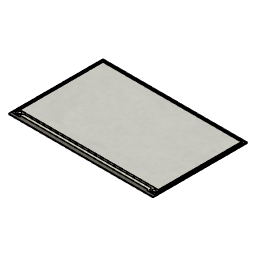
Openbook complet (Autodesk Fusion 360 archive; units mm, degrees)
design "Display"
Autodesk Fusion 360 part; units mm, degrees
sketch "Sketch1" plane through (0, 0, 0) normal (0, 0, 1) x (1, 0, 0)
  line L0 (0, 0) -> (170.2, 0)
  line L1 (170.2, 0) -> (170.2, 111.2)
  line L2 (170.2, 111.2) -> (0, 111.2)
  line L3 (0, 111.2) -> (0, 0)
  dimension "d1" = 170.2
  dimension "d2" = 111.2
  constraint horizontal L0
  constraint vertical L1
  constraint horizontal L2
  constraint vertical L3
  constraint coincident L0.start L3.end
  measures "d1" distance of L0.start L0.end
  measures "d2" distance of L0.end L1.end
extrude "Extrude1" add sketch "Sketch1" along normal blind 0.07 makes body 1
sketch "Sketch2" plane through (0, 0, 0.07) normal (0, 0, 1) x (-1, 0, 0)
  line L0 (0, -111.2) -> (0, 0)
  line L1 (0, 0) -> (-170.2, 0)
  line L2 (-170.2, 0) -> (-170.2, -111.2)
  line L3 (-170.2, -111.2) -> (0, -111.2)
  line L4 (-1.2, -110) -> (-169, -110)
  line L5 (-169, -110) -> (-169, -2.91)
  line L6 (-169, -2.91) -> (-1.2, -2.91)
  line L7 (-1.2, -2.91) -> (-1.2, -110)
  dimension "d6" = 167.8
  dimension "d7" = 107.09
  constraint horizontal L4
  constraint vertical L5
  constraint horizontal L6
  constraint vertical L7
  measures "d6" distance of L4.start L4.end
  measures "d7" distance of L4.start L6.end
extrude "Extrude2" add sketch "Sketch2" along normal blind 0.06 separate body contours L4 L5 L6 L7 makes body 2
sketch "Sketch3" plane through (0, 0, 0.13) normal (0, 0, 1) x (-1, 0, 0)
  line L0 (-1.2, -2.91) -> (-169, -2.91)
  line L1 (-169, -2.91) -> (-169, -110)
  line L2 (-169, -110) -> (-1.2, -110)
  line L3 (-1.2, -110) -> (-1.2, -2.91)
  line L4 (-169, -2.91) -> (-160, -2.91)
  spline S0 degree 5 poles (-10.2, -2.91) (-10.2046, -2.9696) (-10.2134, -3.086) (-10.226, -3.2529) (-10.2412, -3.4594) (-10.258, -3.6905) (-10.2727, -3.8935) (-10.2862, -4.0679) (-10.3001, -4.2136) (-10.3166, -4.3314) (-10.3392, -4.4237) (-10.3718, -4.4938) (-10.4184, -4.5453) (-10.4822, -4.5814) (-10.565, -4.6046) (-10.6676, -4.6167) (-10.7655, -4.6183) (-10.8476, -4.6151) (-10.9061, -4.6111) (-10.9364, -4.6086) knots 0 0 0 0 0 0 0.066667 0.133333 0.2 0.266667 0.333333 0.4 0.466667 0.533333 0.6 0.666667 0.733333 0.8 0.866667 0.933333 1 1 1 1 1 1
  spline S1 degree 5 poles (-160, -2.91) (-160.0003, -2.9773) (-159.9997, -3.108) (-159.9949, -3.2923) (-159.9808, -3.5144) (-159.9499, -3.7519) (-159.9052, -3.9484) (-159.8458, -4.1039) (-159.7711, -4.2198) (-159.6803, -4.3001) (-159.5732, -4.351) (-159.4493, -4.3798) (-159.3085, -4.3938) (-159.1511, -4.3991) (-158.9775, -4.3996) (-158.7883, -4.3978) (-158.625, -4.3954) (-158.4959, -4.3933) (-158.407, -4.3917) (-158.3618, -4.3909) knots 0 0 0 0 0 0 0.066667 0.133333 0.2 0.266667 0.333333 0.4 0.466667 0.533333 0.6 0.666667 0.733333 0.8 0.866667 0.933333 1 1 1 1 1 1
  line L5 (-10.9364, -4.6086) -> (-158.3618, -4.3909)
  point P0 (-10.3, -4.2)
  point P1 (-10.4443, -4.5566)
  point P2 (-159.805, -4.1594)
  point P3 (-159.3149, -4.3909)
  dimension "d10" = 9
  dimension "d11" = 9
  constraint horizontal L4
  constraint coincident L0.end L1.start
  measures "d10" distance of L0.start S0.start
  measures "d11" distance of L0.end L4.end
extrude "Extrude3" cut sketch "Sketch3" against normal blind 0.06 contours L0 S0 S1 L5 bodies 2
sketch "Sketch4" plane through (0, 0, 0.13) normal (0, 0, 1) x (-1, 0, 0)
  spline S0 degree 5 poles (-158.3618, -4.3909) (-158.407, -4.3917) (-158.4959, -4.3933) (-158.625, -4.3954) (-158.7883, -4.3978) (-158.9775, -4.3996) (-159.1511, -4.3991) (-159.3085, -4.3938) (-159.4493, -4.3798) (-159.5732, -4.351) (-159.6803, -4.3001) (-159.7711, -4.2198) (-159.8458, -4.1039) (-159.9052, -3.9484) (-159.9499, -3.7519) (-159.9808, -3.5144) (-159.9949, -3.2923) (-159.9997, -3.108) (-160.0003, -2.9773) (-160, -2.91) knots -1 -1 -1 -1 -1 -1 -0.933333 -0.866667 -0.8 -0.733333 -0.666667 -0.6 -0.533333 -0.466667 -0.4 -0.333333 -0.266667 -0.2 -0.133333 -0.066667 0 0 0 0 0 0
  line L0 (-160, -2.91) -> (-169, -2.91)
  line L1 (-169, -2.91) -> (-169, -110)
  line L2 (-169, -110) -> (-1.2, -110)
  line L3 (-1.2, -110) -> (-1.2, -2.91)
  line L4 (-1.2, -2.91) -> (-10.2, -2.91)
  spline S1 degree 5 poles (-10.2, -2.91) (-10.2046, -2.9696) (-10.2134, -3.086) (-10.226, -3.2529) (-10.2412, -3.4594) (-10.258, -3.6905) (-10.2727, -3.8935) (-10.2862, -4.0679) (-10.3001, -4.2136) (-10.3166, -4.3314) (-10.3392, -4.4237) (-10.3718, -4.4938) (-10.4184, -4.5453) (-10.4822, -4.5814) (-10.565, -4.6046) (-10.6676, -4.6167) (-10.7655, -4.6183) (-10.8476, -4.6151) (-10.9061, -4.6111) (-10.9364, -4.6086) knots 0 0 0 0 0 0 0.066667 0.133333 0.2 0.266667 0.333333 0.4 0.466667 0.533333 0.6 0.666667 0.733333 0.8 0.866667 0.933333 1 1 1 1 1 1
  line L5 (-10.9364, -4.6086) -> (-158.3618, -4.3909)
  line L6 (-2.7, -108.5) -> (-167.5, -108.5)
  line L7 (-167.5, -108.5) -> (-167.5, -4.41)
  line L8 (-167.5, -4.41) -> (-2.7, -4.41)
  line L9 (-2.7, -4.41) -> (-2.7, -108.5)
  dimension "d17" = 164.8
  dimension "d18" = 104.09
  constraint horizontal L6
  constraint vertical L7
  constraint horizontal L8
  constraint vertical L9
  measures "d17" distance of L6.start L6.end
  measures "d18" distance of L6.start L8.end
extrude "Extrude4" add sketch "Sketch4" along normal blind 0.16 separate body contours S1 L5 L6 L7 L8 L9 makes body 3
sketch "Sketch5" plane through (0, 0, 0.07) normal (0, 0, 1) x (-1, 0, 0)
  line L0 (0, -111.2) -> (0, 0)
  line L1 (0, 0) -> (-170.2, 0)
  line L2 (-170.2, 0) -> (-170.2, -111.2)
  line L3 (-170.2, -111.2) -> (0, -111.2)
  line L4 (0, -111.2) -> (-170.2, -111.2)
  line L5 (-170.2, -111.2) -> (-170.2, 0)
  line L6 (-170.2, 0) -> (0, 0)
  line L7 (0, 0) -> (0, -111.2)
  dimension "d21" = 170.2
  dimension "d22" = 111.2
  constraint horizontal L4
  constraint vertical L5
  constraint horizontal L6
  constraint vertical L7
  constraint coincident L0.start L3.end
  measures "d21" distance of L0.start L2.end
  measures "d22" distance of L0.start L0.end
extrude "Extrude5" add sketch "Sketch5" along normal blind 0.63 bodies 1
move_body "Move1" bodies 2 to x (1, 0, 0) y (0, 1, 0) z (0, 0, 1) at (0, 0, 0.7)
extrude "Extrude6" add 1 faces at (109.5206, 74.797, 0.83) along direction (0, 0, 1) blind 0.1 on bodies 2 bodies 2
move_body "Move2" bodies 3 to x (1, 0, 0) y (0, 1, 0) z (0, 0, 1) at (0, 0, 0.86)
sketch "Sketch6" plane through (0, 0, 1.15) normal (0, 0, 1) x (-1, 0, 0)
  spline S0 degree 5 poles (-10.339, -4.41) (-10.3395, -4.4117) (-10.3455, -4.4299) (-10.3581, -4.4622) (-10.3802, -4.5031) (-10.4184, -4.5453) (-10.4822, -4.5814) (-10.565, -4.6046) (-10.6676, -4.6167) (-10.7655, -4.6183) (-10.8476, -4.6151) (-10.9061, -4.6111) (-10.9364, -4.6086) knots 0.526762 0.526762 0.526762 0.526762 0.526762 0.526762 0.533333 0.6 0.666667 0.733333 0.8 0.866667 0.933333 1 1 1 1 1 1
  line L0 (-10.9364, -4.6086) -> (-145.4015, -4.41)
  line L1 (-145.4015, -4.41) -> (-167.5, -4.41)
  line L2 (-167.5, -4.41) -> (-167.5, -108.5)
  line L3 (-167.5, -108.5) -> (-2.7, -108.5)
  line L4 (-2.7, -108.5) -> (-2.7, -4.41)
  line L5 (-2.7, -4.41) -> (-10.339, -4.41)
  spline S1 degree 5 poles (-8.7, -4.41) (-8.707, -4.4556) (-8.7209, -4.5443) (-8.7408, -4.6698) (-8.7659, -4.8221) (-8.7948, -4.9867) (-8.8215, -5.125) (-8.8466, -5.237) (-8.8716, -5.3232) (-8.8985, -5.3859) (-8.9302, -5.4287) (-8.97, -5.4564) (-9.021, -5.4735) (-9.0857, -5.484) (-9.1653, -5.4907) (-9.2604, -5.4952) (-9.3487, -5.4977) (-9.4217, -5.499) (-9.4734, -5.4997) (-9.5, -5.5) knots 0 0 0 0 0 0 0.066667 0.133333 0.2 0.266667 0.333333 0.4 0.466667 0.533333 0.6 0.666667 0.733333 0.8 0.866667 0.933333 1 1 1 1 1 1
  spline S2 degree 5 poles (-161.5, -4.41) (-161.4999, -4.4539) (-161.4995, -4.5394) (-161.4982, -4.6608) (-161.4948, -4.8087) (-161.4879, -4.97) (-161.478, -5.1071) (-161.4646, -5.2198) (-161.4468, -5.3086) (-161.4236, -5.3751) (-161.3936, -5.4225) (-161.3554, -5.4547) (-161.3075, -5.4756) (-161.2488, -5.4889) (-161.179, -5.4968) (-161.0979, -5.501) (-161.0241, -5.5019) (-160.9639, -5.5014) (-160.9217, -5.5006) (-160.9, -5.5) knots 0 0 0 0 0 0 0.066667 0.133333 0.2 0.266667 0.333333 0.4 0.466667 0.533333 0.6 0.666667 0.733333 0.8 0.866667 0.933333 1 1 1 1 1 1
  line L6 (-160.9, -5.5) -> (-9.5, -5.5)
  point P0 (-8.8643, -5.2936)
  point P1 (-9.0307, -5.4733)
  point P2 (-161.451, -5.2805)
  point P3 (-161.2937, -5.4771)
  dimension "d27" = 6
  dimension "d29" = 6
  measures "d27" distance of L4.end S1.start
  measures "d29" distance of L1.end S2.start
extrude "Extrude7" cut sketch "Sketch6" against normal blind 0.16 contours S0 L0 L1 L5 S1 S2 L6 bodies 3
sketch "Sketch7" plane through (0, 0, 1.15) normal (0, 0, 1) x (-1, 0, 0)
  spline S0 degree 5 poles (-160.9, -5.5) (-160.9217, -5.5006) (-160.9639, -5.5014) (-161.0241, -5.5019) (-161.0979, -5.501) (-161.179, -5.4968) (-161.2488, -5.4889) (-161.3075, -5.4756) (-161.3554, -5.4547) (-161.3936, -5.4225) (-161.4236, -5.3751) (-161.4468, -5.3086) (-161.4646, -5.2198) (-161.478, -5.1071) (-161.4879, -4.97) (-161.4948, -4.8087) (-161.4982, -4.6608) (-161.4995, -4.5394) (-161.4999, -4.4539) (-161.5, -4.41) knots -1 -1 -1 -1 -1 -1 -0.933333 -0.866667 -0.8 -0.733333 -0.666667 -0.6 -0.533333 -0.466667 -0.4 -0.333333 -0.266667 -0.2 -0.133333 -0.066667 0 0 0 0 0 0
  line L0 (-161.5, -4.41) -> (-167.5, -4.41)
  line L1 (-167.5, -4.41) -> (-167.5, -108.5)
  line L2 (-167.5, -108.5) -> (-2.7, -108.5)
  line L3 (-2.7, -108.5) -> (-2.7, -4.41)
  line L4 (-2.7, -4.41) -> (-8.7, -4.41)
  spline S1 degree 5 poles (-8.7, -4.41) (-8.707, -4.4556) (-8.7209, -4.5443) (-8.7408, -4.6698) (-8.7659, -4.8221) (-8.7948, -4.9867) (-8.8215, -5.125) (-8.8466, -5.237) (-8.8716, -5.3232) (-8.8985, -5.3859) (-8.9302, -5.4287) (-8.97, -5.4564) (-9.021, -5.4735) (-9.0857, -5.484) (-9.1653, -5.4907) (-9.2604, -5.4952) (-9.3487, -5.4977) (-9.4217, -5.499) (-9.4734, -5.4997) (-9.5, -5.5) knots 0 0 0 0 0 0 0.066667 0.133333 0.2 0.266667 0.333333 0.4 0.466667 0.533333 0.6 0.666667 0.733333 0.8 0.866667 0.933333 1 1 1 1 1 1
  line L5 (-9.5, -5.5) -> (-160.9, -5.5)
  circle A0 centre (-6, -7) radius 1.8477
  circle A1 centre (-164.4622, -6.8748) radius 1.7327
sketch "Sketch8" plane through (0, 0, 1.15) normal (0, 0, 1) x (1, 0, 0)
  line L0 (2.7, 108.5) -> (3.5, 108.5)
  line L1 (3.5, 108.5) -> (3.5, 107.7)
  line L2 (3.5, 107.7) -> (2.7, 107.7)
  line L3 (2.7, 107.7) -> (2.7, 108.5)
  line L4 (3.5, 107.7) -> (166.7, 107.7)
  line L5 (166.7, 107.7) -> (166.7, 9.78)
  line L6 (166.7, 9.78) -> (3.5, 9.78)
  line L7 (3.5, 9.78) -> (3.5, 107.7)
  dimension "d36" = 0.8
  dimension "d37" = 0.8
  dimension "d38" = 163.2
  dimension "d39" = 97.92
  constraint horizontal L0
  constraint vertical L1
  constraint horizontal L2
  constraint vertical L3
  constraint horizontal L4
  constraint vertical L5
  constraint horizontal L6
  constraint vertical L7
  measures "d36" distance of L0.start L0.end
  measures "d37" distance of L0.start L2.end
  measures "d38" distance of L1.end L4.end
  measures "d39" distance of L1.end L6.end
extrude "Extrude8" cut sketch "Sketch7" against normal blind 0.08 contours A0 | A1 bodies 3
extrude "Extrude9" add sketch "Sketch8" along normal blind 0.16 separate body contours L4 L5 L6 L7 makes body 4
sketch "Sketch9" plane through (0, 0, 1.15) normal (0, 0, 1) x (-1, 0, 0)
  circle A0 centre (-6, -7) radius 1.8477
  circle A1 centre (-164.4622, -6.8748) radius 1.7327
  spline S0 degree 5 poles (-160.9, -5.5) (-160.9217, -5.5006) (-160.9639, -5.5014) (-161.0241, -5.5019) (-161.0979, -5.501) (-161.179, -5.4968) (-161.2488, -5.4889) (-161.3075, -5.4756) (-161.3554, -5.4547) (-161.3936, -5.4225) (-161.4236, -5.3751) (-161.4468, -5.3086) (-161.4646, -5.2198) (-161.478, -5.1071) (-161.4879, -4.97) (-161.4948, -4.8087) (-161.4982, -4.6608) (-161.4995, -4.5394) (-161.4999, -4.4539) (-161.5, -4.41) knots -1 -1 -1 -1 -1 -1 -0.933333 -0.866667 -0.8 -0.733333 -0.666667 -0.6 -0.533333 -0.466667 -0.4 -0.333333 -0.266667 -0.2 -0.133333 -0.066667 0 0 0 0 0 0
  line L0 (-161.5, -4.41) -> (-167.5, -4.41)
  line L1 (-167.5, -4.41) -> (-167.5, -108.5)
  line L2 (-167.5, -108.5) -> (-2.7, -108.5)
  line L3 (-2.7, -108.5) -> (-2.7, -4.41)
  line L4 (-2.7, -4.41) -> (-8.7, -4.41)
  spline S1 degree 5 poles (-8.7, -4.41) (-8.707, -4.4556) (-8.7209, -4.5443) (-8.7408, -4.6698) (-8.7659, -4.8221) (-8.7948, -4.9867) (-8.8215, -5.125) (-8.8466, -5.237) (-8.8716, -5.3232) (-8.8985, -5.3859) (-8.9302, -5.4287) (-8.97, -5.4564) (-9.021, -5.4735) (-9.0857, -5.484) (-9.1653, -5.4907) (-9.2604, -5.4952) (-9.3487, -5.4977) (-9.4217, -5.499) (-9.4734, -5.4997) (-9.5, -5.5) knots 0 0 0 0 0 0 0.066667 0.133333 0.2 0.266667 0.333333 0.4 0.466667 0.533333 0.6 0.666667 0.733333 0.8 0.866667 0.933333 1 1 1 1 1 1
  line L5 (-9.5, -5.5) -> (-160.9, -5.5)
  spline S2 degree 5 poles (-8.7, -4.41) (-8.6993, -4.5358) (-8.7019, -4.7829) (-8.7177, -5.1397) (-8.7631, -5.5872) (-8.8631, -6.0966) (-9.0107, -6.551) (-9.2101, -6.9453) (-9.4647, -7.2759) (-9.7735, -7.5438) (-10.1329, -7.753) (-10.4579, -7.8771) (-10.7214, -7.9473) (-10.9057, -7.9841) (-11, -8) knots 0 0 0 0 0 0 0.1 0.2 0.3 0.4 0.5 0.6 0.7 0.8 0.9 1 1 1 1 1 1
  spline S3 degree 5 poles (-161.4997, -4.4901) (-161.5085, -4.5917) (-161.5235, -4.7907) (-161.538, -5.0769) (-161.5412, -5.4335) (-161.5177, -5.8367) (-161.4657, -6.1962) (-161.3845, -6.5109) (-161.2738, -6.7809) (-161.1344, -7.008) (-160.9682, -7.1961) (-160.7777, -7.3502) (-160.5659, -7.4756) (-160.3353, -7.5773) (-160.0882, -7.659) (-159.826, -7.7231) (-159.605, -7.7616) (-159.4332, -7.7836) (-159.316, -7.7952) (-159.2567, -7.8003) knots 0 0 0 0 0 0 0.066667 0.133333 0.2 0.266667 0.333333 0.4 0.466667 0.533333 0.6 0.666667 0.733333 0.8 0.866667 0.933333 1 1 1 1 1 1
  line L6 (-159.2567, -7.8003) -> (-11, -8)
  point P0 (-9.2836, -7.0199)
  point P1 (-161.3, -6.7)
  point P2 (-160.5, -7.5)
  constraint coincident L4.end S1.start
  constraint coincident S0 S3.start
extrude "Extrude10" cut sketch "Sketch9" against normal blind 0.16 contours S0 S1 L5 S2 S3 L6 bodies 3
